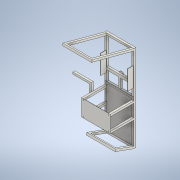
# Autodesk Inventor part: rama pod fotel v2
Saved by Autodesk Inventor 2021 (Build 250183000, 183)
## iProperties
Created: 2022-04-14
Part Number: rama pod fotel v2
Material: Generic
Document SubType Name: Modeling
Designer: Łukasz
Density: 1 g/cm^3
Appearance: Steel
Author: Łukasz
Autodesk Inventor part; units mm, degrees
ref_plane "YZ Plane" through (0, 0, 0) normal (1, 0, 0) x (0, 1, 0)
ref_plane "XZ Plane" through (0, 0, 0) normal (0, 1, 0) x (-1, 0, 0)
ref_plane "XY Plane" through (0, 0, 0) normal (0, 0, 1) x (1, 0, 0)
sketch "Sketch1" plane through (0, 0, 0) normal (0, 0, 1) x (1, 0, 0)
  line L0 (0, 0) -> (-375, 0)
  line L1 (-375, 0) -> (-375, -600)
  line L2 (-375, -600) -> (0, -600)
  line L3 (0, -600) -> (0, 0)
  line L4 (-405, 30) -> (30, 30)
  line L5 (30, 30) -> (30, -630)
  line L6 (30, -630) -> (-405, -630)
  line L7 (-405, -630) -> (-405, 30)
  line L8 (-405, -630) -> (-375, -630)
  line L9 (-375, -630) -> (-375, -1270)
  line L10 (-375, -1270) -> (-405, -1270)
  line L11 (-405, -1270) -> (-405, -630)
  line L12 (30, -630) -> (0, -630)
  line L13 (0, -630) -> (0, -1270)
  line L14 (0, -1270) -> (30, -1270)
  line L15 (30, -1270) -> (30, -630)
  line L16 (-375, -1270) -> (0, -1270)
  line L17 (0, -1270) -> (0, -1240)
  line L18 (0, -1240) -> (-375, -1240)
  line L19 (-375, -1240) -> (-375, -1270)
  dimension "d0" = 375
  dimension "d1" = 600
  dimension "d2" = 30
  dimension "d3" = 30
  dimension "d4" = 30
  dimension "d5" = 30
  dimension "d38" = 30
  dimension "d39" = 640
  dimension "d40" = 30
  dimension "d41" = 640
  dimension "d42" = 30
  constraints: 40 end point, 10 parallel, 5 horizontal, 5 perpendicular, 1 point on line
  measures "d0" distance of L2.end L1.end
  measures "d1" distance of L1.end L0.end
  measures "d2" distance between parallel lines of L4 L0
  measures "d3" distance between parallel lines of L2 L6
  measures "d4" distance between parallel lines of L3 L5
  measures "d5" distance between parallel lines of L1 L7
  measures "d38" distance of L9.end L10.end
  measures "d39" distance of L8.end L9.end
  measures "d40" distance of L14.end L13.end
  measures "d41" distance of L13.end L12.end
  measures "d42" distance of L17.end L16.end
extrude "Extrusion1" add sketch "Sketch1" along normal blind 30 contours L4 L5 L6 L7
sketch "Sketch2" plane through (0, 0, 0) normal (0, 0, -1) x (-1, 0, 0)
  line L0 (375, -600) -> (375, 0) projected
  line L1 (375, -450) -> (0, -450)
  line L2 (0, -450) -> (0, -410)
  line L3 (0, -410) -> (375, -410)
  line L4 (375, -410) -> (375, -450)
  line L5 (0, -600) -> (375, -600) projected
  line L6 (202.5, -600) -> (202.5, -450)
  line L7 (172.5, -600) -> (172.5, -450)
  point P0 (0, 0)
  dimension "d8" = 375
  dimension "d9" = 40
  dimension "d10" = 150
  constraints: 12 end point, 5 point on line, 3 perpendicular, 2 parallel, 1 horizontal
  measures "d8" distance of L2.end L3.end
  measures "d9" distance of L1.end L2.end
  measures "d10" distance between parallel lines of L5 L1
extrude "Extrusion2" add sketch "Sketch2" against normal blind 30 contours L1 L2 L3 L0 | L5 L7 L1 L6
sketch "Sketch3" plane through (0, 0, 30) normal (0, 0, 1) x (1, 0, 0)
  line L0 (12.5, -490) -> (17.5, -490)
  line L1 (17.5, -490) -> (17.5, -200)
  line L2 (17.5, -200) -> (12.5, -200)
  line L3 (12.5, -200) -> (12.5, -490)
  line L4 (0, -410) -> (-375, -410) projected
  line L5 (-392.5, -490) -> (-387.5, -490)
  line L6 (-387.5, -490) -> (-387.5, -200)
  line L7 (-387.5, -200) -> (-392.5, -200)
  line L8 (-392.5, -200) -> (-392.5, -490)
  line L9 (0, -600) -> (-172.5, -600) projected
  point P0 (0, 0)
  dimension "d13" = 5
  dimension "d14" = 290
  dimension "d18" = 405
  dimension "d37" = 110
  constraints: 16 end point, 2 horizontal, 2 parallel, 1 perpendicular, 8 other
  measures "d13" distance of L2.end L1.end
  measures "d14" distance of L1.end L0.end
  measures "d18" distance of L0.start L5.start
  measures "d37" distance from line of L9 L0.start
extrude "Extrusion3" add sketch "Sketch3" along normal blind 80
sketch "Sketch4" plane through (30, -630, 0) normal (1, 0, 0) x (0, 0, -1)
  line L0 (-30, 0) -> (-30, 660) projected
  line L1 (-30, 660) -> (-657.8518, 828.2324)
  line L2 (-30, 660) -> (620, 660) construction
  line L3 (-657.8518, 828.2324) -> (-665.6164, 799.2546)
  line L4 (-665.6164, 799.2546) -> (-30, 628.9417)
  point P0 (0, 630)
  dimension "d25" = 650
  dimension "d26" = 165
  dimension "d27" = 30
  dimension "d28" = 270
  constraints: 8 end point, 2 perpendicular, 1 equal length, 1 horizontal, 1 point on line
  measures "d25" distance of L0.end L1.end
  measures "d26" angle of L2 L1
  measures "d27" distance of L1.end L3.end
extrude "Extrusion4" add sketch "Sketch4" against normal blind 30
pattern_linear "Rectangular Pattern1" count 2 spacing 405 along (-1, 0, 0) of "Extrusion4"
sketch "Sketch5" plane through (-375, 0, 30) normal (1, 0, 0) x (0, 0, -1)
  line L0 (-635.6164, 169.2546) -> (-627.8518, 198.2324) projected
  line L1 (0, -1.0583) -> (-635.6164, 169.2546) projected
  line L2 (-627.8518, 198.2324) -> (-635.6164, 169.2546)
  line L3 (-635.6164, 169.2546) -> (-606.6386, 161.49)
  line L4 (-606.6386, 161.49) -> (-598.874, 190.4678)
  line L5 (-627.8518, 198.2324) -> (0, 30) projected
  line L6 (-627.8518, 198.2324) -> (-598.874, 190.4678)
  point P0 (30, 0)
  dimension "d34" = 30
  constraints: 8 end point, 3 perpendicular, 2 point on line
  measures "d34" distance of L0.start L3.end
extrude "Extrusion5" add sketch "Sketch5" along normal up to surface (375 mm away)
sketch "Sketch6" plane through (0, 0, 0) normal (0, 0, -1) x (-1, 0, 0)
  line L0 (0, -630) -> (0, -1270)
  line L1 (0, -1270) -> (-30, -1270)
  line L2 (-30, -1270) -> (-30, -630)
  line L3 (375, -630) -> (375, -1270)
  line L4 (375, -1270) -> (405, -1270)
  line L5 (405, -1270) -> (405, -630)
  line L6 (0, -1270) -> (375, -1270)
  line L7 (375, -1270) -> (375, -1240)
  line L8 (375, -1240) -> (0, -1240)
  line L9 (0, -1240) -> (0, -1270)
  line L10 (405, -1.0583) -> (405, -630) projected
  line L11 (-30, -630) -> (-30, -1.0583) projected
  line L12 (405, -630) -> (375, -630)
  line L13 (405, -630) -> (-30, -630) projected
  line L14 (0, -630) -> (-30, -630)
  point P0 (0, 0)
  dimension "d43" = 30
  dimension "d44" = 640
  dimension "d45" = 30
  dimension "d46" = 640
  dimension "d47" = 30
  dimension "d48" = 0
  dimension "d49" = 0
  constraints: 24 end point, 4 parallel, 2 collinear, 1 horizontal, 1 perpendicular, 1 point on line
  measures "d43" distance of L1.start L1.end
  measures "d44" distance of L0.start L1.start
  measures "d45" distance of L4.end L4.start
  measures "d46" distance of L4.start L3.start
  measures "d47" distance of L8.start L6.end
  measures "d48" distance between parallel lines of L10 L5
  measures "d49" distance between parallel lines of L11 L2
extrude "Extrusion6" add sketch "Sketch6" against normal blind 30 contours L0 L1 L2 L13 | L8 L3 L6 L0 | L12 L5 L4 L3
sketch "Sketch7" plane through (0, 0, 0) normal (0, 0, -1) x (-1, 0, 0)
  circle A0 centre (187.5, -430) radius 40
  point P0 (0, 0)
  dimension "d52" = 80
  constraints: 1 centre point
  measures "d52" diameter of A0
extrude "Extrusion7" add sketch "Sketch7" along normal blind 5 and the other way blind 5
sketch "Sketch8" plane through (30, -1270, 0) normal (1, 0, 0) x (0, 0, -1)
  line L0 (0, 0) -> (-30, 0) projected
  line L1 (-30, 0) -> (-311.9078, 102.606)
  line L2 (-30, 0) -> (270, 0) construction
  line L3 (-311.9078, 102.606) -> (-301.6472, 130.7968)
  line L4 (-301.6472, 130.7968) -> (-30, 31.9253)
  line L5 (-30, 640) -> (-30, 30) projected
  line L6 (-30, 31.9253) -> (-30, 0)
  point P0 (0, 1270)
  dimension "d55" = 300
  dimension "d56" = 160
  dimension "d57" = 30
  dimension "d58" = 90
  constraints: 10 end point, 1 equal length, 1 horizontal, 1 perpendicular, 1 point on line, 1 vertical
  measures "d55" distance of L0.end L1.end
  measures "d56" angle of L2 L1
  measures "d57" distance of L1.end L3.end
  measures "d58" angle of L3 L4
extrude "Extrusion8" add sketch "Sketch8" against normal blind 30
pattern_linear "Rectangular Pattern2" count 2 spacing 405 along (-1, 0, 0) of "Extrusion8"
sketch "Sketch9" plane through (0, -1240, 0) normal (-1, 0, 0) x (0, 0, 1)
  line L0 (311.9078, 72.606) -> (301.6472, 100.7968) projected
  line L1 (311.9078, 72.606) -> (301.6472, 100.7968)
  line L2 (301.6472, 100.7968) -> (273.4564, 90.5362)
  line L3 (30, 1.9253) -> (301.6472, 100.7968) projected
  line L4 (273.4564, 90.5362) -> (283.717, 62.3454)
  line L5 (30, -30) -> (311.9078, 72.606) projected
  line L6 (283.717, 62.3454) -> (311.9078, 72.606)
  point P0 (0, 1240)
  dimension "d64" = 30
  constraints: 8 end point, 2 perpendicular, 1 collinear, 1 point on line
  measures "d64" distance of L0.end L2.end
extrude "Extrusion9" add sketch "Sketch9" along normal up to surface (375 mm away)
sketch "Sketch10" plane through (0, 0, 30) normal (0, 0, 1) x (1, 0, 0)
  line L0 (-405, -1238.0747) -> (-375, -1238.0747) projected
  line L1 (-405, -1238.0747) -> (30, -1238.0747)
  line L2 (30, -1238.0747) -> (30, -598.0747)
  line L3 (30, -598.0747) -> (-405, -598.0747)
  line L4 (-405, -598.0747) -> (-405, -1238.0747)
  point P0 (0, 0)
  dimension "d67" = 435
  dimension "d68" = 640
  constraints: 8 end point, 2 parallel, 1 horizontal, 1 perpendicular
  measures "d67" distance of L3.end L2.end
  measures "d68" distance of L2.end L1.end
extrude "Extrusion10" add sketch "Sketch10" along normal blind 2
sketch "Sketch11" plane through (0, 0, 32) normal (0, 0, 1) x (1, 0, 0)
  line L0 (30, -648.0747) -> (0, -648.0747)
  line L1 (0, -648.0747) -> (0, -678.0747)
  line L2 (0, -678.0747) -> (30, -678.0747)
  line L3 (30, -678.0747) -> (30, -648.0747)
  line L4 (30, -598.0747) -> (-405, -598.0747) projected
  point P0 (0, 0)
  dimension "d71" = 30
  dimension "d72" = 30
  dimension "d73" = 50
  constraints: 8 end point, 2 parallel, 1 horizontal, 1 perpendicular
  measures "d71" distance of L2.end L1.end
  measures "d72" distance of L1.end L0.end
  measures "d73" distance between parallel lines of L4 L0
extrude "Extrusion11" add sketch "Sketch11" along normal blind 350
pattern_linear "Rectangular Pattern3" count 2 spacing 220 along (0, -1, 0) count 2 spacing 405 along (-1, 0, 0) of "Extrusion11"
sketch "Sketch12" plane through (0, 0, 382) normal (0, 0, 1) x (1, 0, 0)
  line L0 (-405, -868.0747) -> (-405, -898.0747) projected
  line L1 (-405, -898.0747) -> (-375, -898.0747) projected
  line L2 (-375, -898.0747) -> (-375, -868.0747) projected
  line L3 (-375, -868.0747) -> (-405, -868.0747) projected
  line L4 (-405, -648.0747) -> (-405, -678.0747) projected
  line L5 (-405, -678.0747) -> (-375, -678.0747) projected
  line L6 (-375, -678.0747) -> (-375, -648.0747) projected
  line L7 (-375, -648.0747) -> (-405, -648.0747) projected
  line L8 (0, -648.0747) -> (0, -678.0747) projected
  line L9 (0, -678.0747) -> (30, -678.0747) projected
  line L10 (30, -678.0747) -> (30, -648.0747) projected
  line L11 (30, -648.0747) -> (0, -648.0747) projected
  line L12 (0, -868.0747) -> (0, -898.0747) projected
  line L13 (0, -898.0747) -> (30, -898.0747) projected
  line L14 (30, -898.0747) -> (30, -868.0747) projected
  line L15 (30, -868.0747) -> (0, -868.0747) projected
  line L16 (-405, -898.0747) -> (-375, -898.0747) projected
  line L17 (-405, -898.0747) -> (30, -898.0747)
  line L18 (30, -898.0747) -> (30, -648.0747)
  line L19 (30, -648.0747) -> (-405, -648.0747)
  line L20 (-405, -648.0747) -> (-405, -898.0747)
  point P0 (0, 0)
  point P1 (0, -898.0747)
  point P2 (30, -868.0747)
  point P3 (30, -678.0747)
  point P4 (0, -648.0747)
  constraints: 8 end point, 2 parallel, 1 horizontal, 1 perpendicular
extrude "Extrusion12" add sketch "Sketch12" against normal blind 3 contours L20 L5 L6 L19 L8 L9 L18 L15 L12 L17 L2 L3
sketch "Sketch13" plane through (-405, -1270, 0) normal (-1, 0, 0) x (0, 0, 1)
  line L0 (232, 591.9253) -> (202, 591.9253)
  line L1 (202, 591.9253) -> (202, 741.9253)
  line L2 (202, 741.9253) -> (232, 741.9253)
  line L3 (232, 741.9253) -> (232, 591.9253)
  line L4 (32, 591.9253) -> (379, 591.9253) projected
  line L5 (382, 621.9253) -> (382, 371.9253) projected
  point P0 (0, 1270)
  dimension "d84" = 30
  dimension "d85" = 150
  dimension "d86" = 0
  dimension "d87" = 150
  constraints: 8 end point, 2 parallel, 1 horizontal, 1 perpendicular
  measures "d84" distance of L1.end L2.end
  measures "d85" distance of L0.end L1.end
  measures "d86" distance between parallel lines of L4 L0
  measures "d87" distance between parallel lines of L5 L3
extrude "Extrusion13" add sketch "Sketch13" along normal blind 30
sketch "Sketch14" plane through (-435, -1270, 0) normal (-1, 0, 0) x (0, 0, 1)
  line L0 (232, 741.9253) -> (202, 741.9253) projected
  line L1 (232, 741.9253) -> (202, 741.9253)
  line L2 (202, 741.9253) -> (202, 711.9253)
  line L3 (202, 711.9253) -> (232, 711.9253)
  line L4 (232, 711.9253) -> (232, 741.9253)
  point P0 (0, 1270)
  point P1 (202, 741.9253)
  dimension "d90" = 30
  dimension "d91" = 30
  constraints: 8 end point, 2 parallel, 1 horizontal, 1 perpendicular
  measures "d90" distance of L3.end L2.end
  measures "d91" distance of L2.end L1.end
extrude "Extrusion14" add sketch "Sketch14" along normal blind 250
sketch "Sketch15" plane through (30, -1270, 0) normal (1, 0, 0) x (0, 0, -1)
  line L0 (-657.8518, 1468.2324) -> (-665.6164, 1439.2546) construction
  circle A0 centre (-661.7341, 1453.7435) radius 7.5 construction
  circle A1 centre (-654.5905, 1451.4588) radius 4
  point P0 (0, 1270)
  dimension "d96" = 15
  dimension "d97" = 8
  constraints: 1 centre point, 1 midpoint, 3 other
  measures "d97" diameter of A1
extrude "Extrusion15" cut sketch "Sketch15" against normal through all
body "Solid1"
